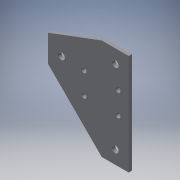
# Autodesk Inventor part: 15102898-16-P-0309
Saved by Autodesk Inventor 2017 (Build 210142000, 142)
## iProperties
Created: 2016-10-08
Part Number: 15102898-16-P-0309
Material: Generic
Document SubType Name: Modeling
Designer: gus
Density: 1 g/cm^3
Appearance: Default
Author: gus
Autodesk Inventor part; units mm, degrees
ref_plane "YZ Plane" through (0, 0, 0) normal (1, 0, 0) x (0, 1, 0)
ref_plane "XZ Plane" through (0, 0, 0) normal (0, 1, 0) x (-1, 0, 0)
ref_plane "XY Plane" through (0, 0, 0) normal (0, 0, 1) x (1, 0, 0)
sketch "Sketch1" plane through (0, 0, 0) normal (0, 0, 1) x (1, 0, 0)
  line L0 (0, 0) -> (50.8, 19.05)
  line L1 (50.8, 19.05) -> (76.2, 19.05)
  line L2 (76.2, 19.05) -> (76.2, -76.2)
  line L3 (76.2, -76.2) -> (50.8, -76.2)
  line L4 (50.8, -76.2) -> (0, -25.4)
  line L5 (0, -25.4) -> (0, 0)
  line L6 (76.2, -6.35) -> (26.8732, -6.35) construction
  line L7 (26.8732, -6.35) -> (26.8732, -41.7576) construction
  line L8 (26.8732, -41.7576) -> (76.2, -41.7576) construction
  line L9 (76.2, -41.7576) -> (76.2, -6.35) construction
  circle A0 centre (33.8732, -13.65) radius 2.3813
  circle A1 centre (66.0064, -13.65) radius 2.3813
  circle A2 centre (33.8732, -34.4576) radius 2.3813
  circle A3 centre (66.0064, -34.4576) radius 2.3813
  line L10 (0, 0) -> (76.2, 0) construction
  circle A4 centre (12.7, -12.7) radius 3.175
  circle A5 centre (63.5, -63.5) radius 3.175
  circle A6 centre (63.5, 6.35) radius 3.175
  dimension "d0" = 25.4
  dimension "d1" = 95.25
  dimension "d2" = 19.05
  dimension "d3" = 76.2
  dimension "d4" = 25.4
  dimension "d5" = 25.4
  dimension "d6" = 49.3268
  dimension "d7" = 35.4076
  dimension "d8" = 25.4
  dimension "d9" = 4.7625
  dimension "d10" = 7.3
  dimension "d11" = 7.3
  dimension "d12" = 7.3
  dimension "d13" = 7.3
  dimension "d14" = 10.1936
  dimension "d15" = 10.1936
  dimension "d16" = 7
  dimension "d17" = 7
  dimension "d18" = 6.35
  dimension "d19" = 12.7
  dimension "d20" = 12.7
  dimension "d21" = 6.35
  dimension "d22" = 6.35
  dimension "d23" = 12.7
  dimension "d24" = 12.7
  dimension "d25" = 12.7
  dimension "d26" = 12.7
  constraints: 22 end point, 7 centre point, 5 perpendicular, 3 equal radius, 2 horizontal, 2 parallel, 2 point on line
  measures "d0" distance of L4.end L0.start
  measures "d1" distance of L1.end L2.end
  measures "d2" distance from line of L0.start L1
  measures "d3" distance between parallel lines of L2 L5
  measures "d4" distance of L0.end L1.end
  measures "d5" distance of L2.end L3.end
  measures "d6" distance of L6.start L6.end
  measures "d7" distance of L6.end L7.end
  measures "d8" distance between parallel lines of L1 L6
  measures "d9" diameter of A2
  measures "d10" distance from line of L6 A0.centre
  measures "d11" distance from line of L6 A1.centre
  measures "d12" distance from line of L8 A2.centre
  measures "d13" distance from line of L8 A3.centre
  measures "d14" distance from line of L2 A3.centre
  measures "d15" distance from line of L2 A1.centre
  measures "d16" distance from line of L7 A0.centre
  measures "d17" distance from line of A2.centre L7
  measures "d18" diameter of A4
  measures "d19" distance from line of L5 A4.centre
  measures "d20" distance from line of L10 A4.centre
  measures "d21" diameter of A6
  measures "d22" diameter of A5
  measures "d23" distance from line of L1 A6.centre
  measures "d24" distance from line of L2 A6.centre
  measures "d25" distance from line of L2 A5.centre
  measures "d26" distance from line of L3 A5.centre
extrude "Extrusion1" add sketch "Sketch1" along normal blind 3.175
body "Solid1"
